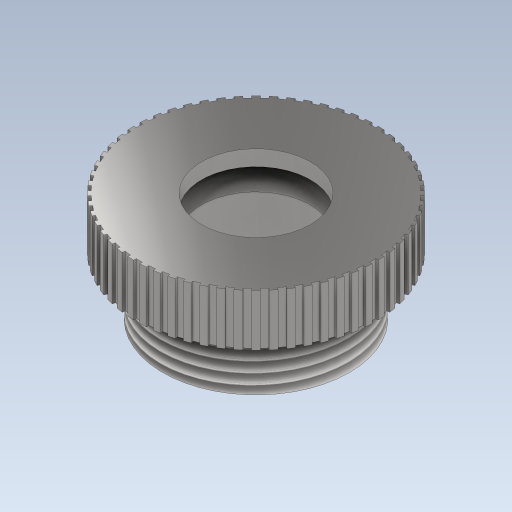
# Autodesk Inventor part: Pump-Motor-CW-Rotation:Cover 102
Saved by Autodesk Inventor 2024.2 (Build 282272000, 272)
## iProperties
Created: 2025-06-16
Material: Steel
Document SubType Name: Modeling
Density: 7.85 g/cm^3
Appearance: Semi-Polished
Designer: cw
Author: cw
Autodesk Inventor part; units mm, degrees
ref_plane "YZ Plane" through (0, 0, 0) normal (1, 0, 0) x (0, 1, 0)
ref_plane "XZ Plane" through (0, 0, 0) normal (0, 1, 0) x (-1, 0, 0)
ref_plane "XY Plane" through (0, 0, 0) normal (0, 0, 1) x (1, 0, 0)
sketch "Sketch1" plane through (0, 0, 0) normal (0, 1, 0) x (-1, 0, 0)
  line L0 (-23, 10.5) -> (0, 10.5)
  line L1 (0, 10.5) -> (0, -10.5)
  line L2 (0, -10.5) -> (-23, -10.5)
  line L3 (-23, -10.5) -> (-23, 10.5)
  line L4 (-23, 0.5) -> (-18, 0.5)
  line L5 (-18, 0.5) -> (-18, -10.5)
  line L6 (-10.5, 10.5) -> (-10.5, -10.5)
  line L7 (-10.5, 7.5) -> (-15.5, 6.9)
  line L8 (-15.5, 6.9) -> (-15.5, 3.9)
  line L9 (-15.5, 3.9) -> (-10.5, 3.3)
  point P0 (0, 0)
  point P1 (0, 0)
  dimension "d0" = 46
  dimension "d1" = 36
  dimension "d2" = 21
  dimension "d3" = 11
  dimension "d4" = 21
  dimension "d5" = 3
  dimension "d6" = 4.2
  dimension "d7" = 31
  dimension "d8" = 3
  constraints: 20 end point, 6 point on line, 3 perpendicular, 2 horizontal, 2 parallel, 1 coincident, 1 equal length, 1 midpoint, 1 vertical
  measures "d0" diameter of L3 L1
  measures "d1" diameter of L5 L1
  measures "d2" distance of L2.end L0.start
  measures "d3" distance between parallel lines of L4 L2
  measures "d4" diameter of L6 L1
  measures "d5" distance from line of L7.start L0
  measures "d6" distance of L9.end L7.start
  measures "d7" diameter of L8 L1
  measures "d8" distance of L7.end L8.end
revolve "Revolution1" add sketch "Sketch1" angle 360 about axis through (0, 0, 10.5) along (0, 0, -1) contours L0 L6 L7 L8 L9 L2 L5 L4 L3
thread "Thread1" size "M36x2" class "6g" standard "ISO Metric profile" length 10
sketch "Sketch2" plane through (0, 0, 10.5) normal (0, 0, 1) x (1, 0, 0)
  line L0 (0, 0) -> (-0.6021, 22.9921)
  circle A0 centre (0, 0) radius 23 projected
  line L1 (0.6021, 22.9921) -> (0, 0)
  arc A1 (0.589, 22.4923) -> (-0.589, 22.4923) centre (0, 0) ccw
  dimension "d12" = 22.5
  dimension "d13" = 3
  constraints: 4 end point, 4 point on circle, 2 point on line, 1 centre point, 1 coincident, 1 horizontal alignment
  measures "d12" radius of A1
  measures "d13" angle of L1 L0
extrude "Extrusion1" cut sketch "Sketch2" against normal through all contours L0 A0 L1 A1
pattern_circular "Circular Pattern1" count 60 over 360 about axis through (0, 0, -10) along (0, 0, 1) of "Extrusion1"
body "Solid1"
